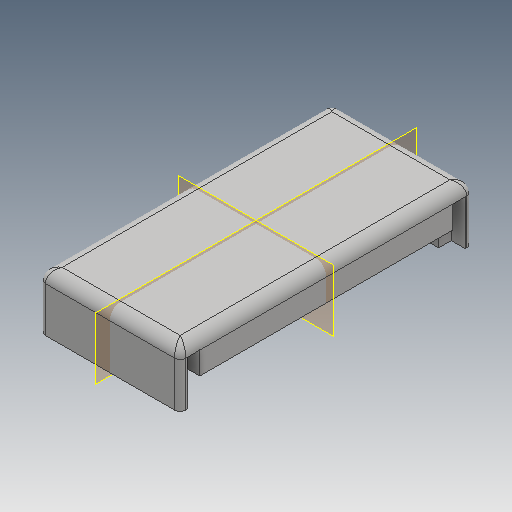
# Autodesk Inventor part: 10x20mm_Cuvette_Bottom
Saved by Autodesk Inventor 2019 (Build 230136000, 136)
## iProperties
Created: 2018-07-25
Part Number: 10x20mm_Cuvette_Bottom
Material: Generic
Document SubType Name: Modeling
Designer: voigt
Density: 1 g/cm^3
Appearance: Default
Author: voigt
Autodesk Inventor part; units mm, degrees
ref_plane "YZ Plane" through (0, 0, 0) normal (1, 0, 0) x (0, 1, 0)
ref_plane "XZ Plane" through (0, 0, 0) normal (0, 1, 0) x (-1, 0, 0)
ref_plane "XY Plane" through (0, 0, 0) normal (0, 0, 1) x (1, 0, 0)
sketch "Sketch1" plane through (0, 0, 0) normal (0, 0, 1) x (1, 0, 0)
  line L0 (6.25, 11.25) -> (-6.25, 11.25) construction
  line L1 (-6.25, 11.25) -> (-6.25, -11.25) construction
  line L2 (-6.25, -11.25) -> (6.25, -11.25) construction
  line L3 (6.25, -11.25) -> (6.25, 11.25) construction
  circle A0 centre (-5.5, -11.875) radius 0.5 construction
  circle A1 centre (-5.5, 11.875) radius 0.5 construction
  circle A2 centre (5.5, 11.875) radius 0.5 construction
  circle A3 centre (5.5, -11.875) radius 0.5 construction
  line L4 (-6.25, 11.25) -> (6.25, 11.25) construction
  line L5 (6.25, 11.25) -> (6.25, -11.25) construction
  line L6 (6.25, -11.25) -> (-6.25, -11.25) construction
  line L7 (-6.25, -11.25) -> (-6.25, 11.25) construction
  line L8 (7.5, -15) -> (7.5, 15) construction
  line L9 (7.5, 15) -> (-7.5, 15) construction
  line L10 (-7.5, 15) -> (-7.5, -15) construction
  line L11 (-7.5, -15) -> (7.5, -15) construction
  line L12 (6.25, 13) -> (-6.25, 13)
  line L13 (-6.25, 13) -> (-6.25, -13)
  line L14 (-6.25, -13) -> (6.25, -13)
  line L15 (6.25, -13) -> (6.25, 13)
  line L16 (-10.5, 0) -> (10.5, 0) construction
  point P0 (0, 0)
  dimension "d0" = 26
  constraints: 8 end point, 2 collinear, 2 parallel, 1 horizontal, 1 perpendicular, 1 other
  measures "d0" distance between parallel lines of L14 L12
extrude "Extrusion1" add sketch "Sketch1" along normal blind 3
sketch "Sketch2" plane through (0, 0, 0) normal (0, 0, -1) x (-1, 0, 0)
  line L0 (-6.25, 13) -> (6.25, 13) construction
  line L1 (-6.25, -13) -> (-6.25, 13) construction
  line L2 (6.25, -13) -> (-6.25, -13) construction
  line L3 (6.25, 13) -> (6.25, -13) construction
  line L4 (-6.25, 11.25) -> (6.25, 11.25) construction
  line L5 (6.25, 11.25) -> (6.25, -11.25) construction
  line L6 (6.25, -11.25) -> (-6.25, -11.25) construction
  line L7 (-6.25, -11.25) -> (-6.25, 11.25) construction
  line L8 (-6.25, 11.25) -> (6.25, 11.25)
  line L9 (6.25, 11.25) -> (6.25, 13)
  line L10 (6.25, 13) -> (-6.25, 13)
  line L11 (-6.25, 13) -> (-6.25, 11.25)
  line L12 (6.25, -13) -> (-6.25, -13) projected
  line L13 (-6.25, -13) -> (6.25, -13)
  line L14 (6.25, -13) -> (6.25, -11.25)
  line L15 (6.25, -11.25) -> (-6.25, -11.25)
  line L16 (-6.25, -11.25) -> (-6.25, -13)
  point P0 (0, 0)
  constraints: 16 end point, 4 parallel, 2 horizontal, 2 perpendicular
extrude "Extrusion2" add sketch "Sketch2" along normal blind 2
sketch "Sketch4" plane through (0, 0, -2) normal (0, 0, -1) x (-1, 0, 0)
  line L0 (-6.25, -13) -> (6.25, -13) construction
  line L1 (6.25, -13) -> (6.25, -11.25) construction
  line L2 (6.25, -11.25) -> (-6.25, -11.25) construction
  line L3 (-6.25, -11.25) -> (-6.25, -13) construction
  line L4 (6.25, 11.25) -> (6.25, 13) construction
  line L5 (6.25, 13) -> (-6.25, 13) construction
  line L6 (-6.25, 13) -> (-6.25, 11.25) construction
  line L7 (-6.25, 11.25) -> (6.25, 11.25) construction
  circle A0 centre (-5.5, -11.875) radius 0.5 construction
  circle A1 centre (-5.5, 11.875) radius 0.5 construction
  circle A2 centre (5.5, 11.875) radius 0.5 construction
  circle A3 centre (5.5, -11.875) radius 0.5 construction
  line L8 (-6.25, -11.25) -> (-5, -11.25)
  line L9 (-5, -11.25) -> (-5, -12.375)
  line L10 (-5, -12.375) -> (-6.25, -12.375)
  line L11 (-6.25, -12.375) -> (-6.25, -11.25)
  point P0 (0, 0)
  point P1 (-5.5, -12.375)
  point P2 (-5.5, -11.375)
  dimension "d19" = 1.125
  dimension "d20" = 1.25
  constraints: 8 end point, 2 parallel, 2 point on circle, 1 horizontal, 1 perpendicular, 1 point on line
  measures "d19" distance between parallel lines of L2 L10
  measures "d20" distance between parallel lines of L11 L9
extrude "Extrusion3" cut sketch "Sketch4" against normal blind 3.5
ref_plane "Work Plane1" through (-6.25, 0, 3) normal (0, -1, 0) x (1, 0, 0)
ref_plane "Work Plane2" through (0, -13, 3) normal (1, 0, 0) x (0, 0, -1)
mirror "Mirror1" about plane through (-6.25, 0, 3) normal (0, -1, 0) of "Extrusion3"
mirror "Mirror2" about plane through (0, -13, 3) normal (1, 0, 0) of "Extrusion3", "Mirror1"
sketch "Sketch5" plane through (-6.25, -11.25, 0) normal (-1, 0, 0) x (0, 0, 1)
  line L0 (0, 22.5) -> (0, 0) construction
  line L1 (3, 24.25) -> (3, -1.75) construction
  line L2 (-2, -1.75) -> (3, -1.75) construction
  line L3 (1.5, -1.125) -> (-2, -1.125) construction
  line L4 (-2, -1.75) -> (-2, -1.125) construction
  line L5 (-2, -1.75) -> (3, -1.75) construction
  line L6 (3, 24.25) -> (3, -1.75) construction
  line L7 (-2, 23.625) -> (1.5, 23.625) construction
  line L8 (3, 24.25) -> (3, -1.75) construction
  line L9 (-2, 24.25) -> (3, 24.25) construction
  line L10 (-2, 23.625) -> (-2, 24.25) construction
  line L11 (0, 0) -> (3, 0) projected
  line L12 (1, 0) -> (2, 0)
  line L13 (2, 0) -> (2, -1.125)
  line L14 (2, -1.125) -> (1, -1.125)
  line L15 (1, -1.125) -> (1, 0)
  line L16 (4, 11.25) -> (-3, 11.25) construction
  line L17 (1.5, 22.5) -> (0, 22.5) projected
  line L18 (0, 22.5) -> (0, 0) projected
  line L19 (0, 0) -> (1.5, 0) projected
  line L20 (1.5, 0) -> (1.5, -1.125) projected
  line L21 (1.5, -1.125) -> (-2, -1.125) projected
  line L22 (-2, -1.75) -> (-2, -1.125) projected
  line L23 (-2, -1.75) -> (3, -1.75) projected
  line L24 (1.5, 23.625) -> (1.5, 22.5) projected
  line L25 (1.5, 22.5) -> (0, 22.5) projected
  line L26 (0, 22.5) -> (0, 0) projected
  line L27 (0, 0) -> (1.5, 0) projected
  line L28 (1.5, 0) -> (1.5, -1.125) projected
  line L29 (-2, 24.25) -> (3, 24.25) projected
  line L30 (-2, 23.625) -> (-2, 24.25) projected
  line L31 (-2, 23.625) -> (1.5, 23.625) projected
  line L32 (1.5, 23.625) -> (1.5, 22.5) projected
  line L33 (1.5, 22.5) -> (0, 22.5) projected
  line L34 (0, 0) -> (1.5, 0) projected
  line L35 (1.5, 0) -> (1.5, -1.125) projected
  line L36 (1.5, -1.125) -> (-2, -1.125) projected
  line L37 (-2, -1.75) -> (-2, -1.125) projected
  line L38 (-2, -1.75) -> (3, -1.75) projected
  line L39 (-2, 24.25) -> (3, 24.25) projected
  line L40 (-2, 23.625) -> (-2, 24.25) projected
  line L41 (-2, 23.625) -> (1.5, 23.625) projected
  line L42 (1.5, 23.625) -> (1.5, 22.5) projected
  point P0 (0, 11.25)
  dimension "d21" = 1
  dimension "d22" = 1
  constraints: 8 end point, 2 parallel, 2 point on line, 1 horizontal, 1 perpendicular
  measures "d21" distance between parallel lines of L15 L13
  measures "d22" distance between parallel lines of L0 L15
extrude "Extrusion4" cut sketch "Sketch5" against normal up to next
mirror "Mirror3" about plane through (-6.25, 0, 3) normal (0, -1, 0) of "Extrusion4"
fillet "Fillet1" radius 1 4 edges at (-5, -11.8125, 1) (-5, 11.8125, 1) (5, 11.8125, 1) (5, -11.8125, 1)
fillet "Fillet3" radius 1 4 edges at (-6.25, 0, 3) (6.25, 0, 3) (0, -13, 3) (0, 13, 3)
fillet "Fillet4" radius 0.5 8 edges at (5.9571, -12.7071, 2.7071) (6.25, -13, 0.0001) (-5.9571, -12.7071, 2.7071) (-6.25, -13, 0.0001) (-5.9571, 12.7071, 2.7071) (-6.25, 13, 0.0001) (5.9571, 12.7071, 2.7071) (6.25, 13, 0.0001)
body "Solid1"
